Toggle Switch - eBay_v1 (Autodesk Fusion 360 design; units mm, degrees)
Autodesk Fusion 360 part; units mm, degrees
sketch "Sketch1" plane through (0, 0, 0) normal (0, 0, 1) x (1, 0, 0)
  line L0 (7.625, -14.5) -> (-7.625, -14.5)
  line L1 (-7.625, -14.5) -> (-7.625, 14.5)
  line L2 (-7.625, 14.5) -> (7.625, 14.5)
  line L3 (7.625, 14.5) -> (7.625, -14.5)
  line L4 (7.625, -14.5) -> (-7.625, 14.5) construction
  line L5 (-7.625, -14.5) -> (7.625, 14.5) construction
  circle A0 centre (0, 0) radius 5.845
  line L6 (-6.335, -5.24) -> (6.335, -5.24)
  arc A1 (6.335, -5.24) -> (6.335, -2.66) centre (6.335, -3.95) ccw
  line L7 (6.335, -2.66) -> (-6.335, -2.66)
  arc A2 (-6.335, -2.66) -> (-6.335, -5.24) centre (-6.335, -3.95) ccw
  line L8 (-7.625, -3.95) -> (7.625, -3.95) construction
  line L9 (0, 0) -> (7.625, 0) construction
  line L10 (6.335, 2.66) -> (-6.335, 2.66)
  arc A3 (-6.335, 5.24) -> (-6.335, 2.66) centre (-6.335, 3.95) ccw
  line L11 (-6.335, 5.24) -> (6.335, 5.24)
  arc A4 (6.335, 2.66) -> (6.335, 5.24) centre (6.335, 3.95) ccw
  dimension "d1" = 15.25
  dimension "d2" = 29
  dimension "d3" = 11.69
  dimension "d6" = 3.95
  dimension "d7" = 2.58
  constraint horizontal L0
  constraint perpendicular L0 L1
  constraint parallel L0 L2
  constraint parallel L1 L3
  constraint coincident L4 A0.centre
  constraint coincident L5 A0.centre
  constraint coincident A0.centre L9.start
  constraint tangent L6 A1
  constraint tangent A1 L7
  constraint parallel L6 L7
  constraint tangent L7 A2
  constraint tangent L6 A2
  constraint midpoint A2 L8.start
  constraint midpoint A1 L8.end
  constraint coincident L3 L8.end
  constraint perpendicular L3 L8
  constraint coincident L1 L8.start
  constraint midpoint L3 L9.end
  constraint symmetric L6.start L9 A3.start
  constraint symmetric L6.end L9 L11.end
  constraint symmetric A1.end L9 L10.start
  constraint symmetric L7.end L9 L10.end
  constraint symmetric A1 L9 A4
  constraint symmetric A2 L9 A3
  measures "d1" distance of L1.end L2.end
  measures "d2" distance of L0.start L2.end
  measures "d3" diameter of A0
  measures "d6" distance of A0.centre L8
  measures "d7" distance of L6 L7
extrude "Extrude1" add sketch "Sketch1" against normal blind 17.25 makes body 1
extrude "Extrude2" add sketch "Sketch1" against normal blind 2 from surface at -17.25 contours A0 L6 A1 L7 | A0 L6 L7 A2 | A0 L10 L11 A4 | A0 L10 A3 L11 | A0 L6 L7 | A0 L10 L11 bodies 1
extrude "Extrude3" add sketch "Sketch1" along normal blind 10.45 contours A0 L6 L7 | A0 L6 | A0 L7 L10 | A0 L10 L11 | A0 L11 bodies 1
thread "Thread1" "ISO Metric profile 12.0 M12x0.5 6g" major diameter 11.927 minor diameter 11.348 pitch 0.5 angle 60 resizes the face on face at (5.816, -0.582, 3.4833) on bodies 1
sketch "Sketch2" plane through (0, 0, 10.45) normal (0, 0, 1) x (-1, 0, 0)
  circle A0 centre (0, 0) radius 5.9635
  circle A1 centre (0, 0) radius 2.25
  dimension "d13" = 4.5
  constraint concentric A0 A1
  measures "d13" diameter of A1
ref_plane "WorkPlane1" through (0, 0, 27.05) normal (0, 0, 1) x (-1, 0, 0)
sketch "Sketch3" plane through (0, 0, 27.05) normal (0, 0, 1) x (1, 0, 0)
  circle A0 centre (0, 0) radius 2.96
  dimension "d15" = 5.92
  constraint coincident A0.centre origin
  measures "d15" diameter of A0
loft "Loft1" add profiles "Sketch2", "Sketch3" section 1 contours A1 section 2 separate body makes body 2
fillet "Fillet1" radius 1.5 1 edges at (-2.7597, 1.0704, 27.05) on bodies 2
move_body "Move1" bodies 2 to x (1, 0, 0) y (0, 0.976296, -0.21644) z (0, 0.21644, 0.976296) at (0, -2.2618, 0.2477)
extrude "Extrude4" add 1 faces at (0.1619, 0.6816, 10.2989) along direction (0, -0.21644, -0.976296) blind 2.5 on bodies 2 bodies 2
equation "d6 = ( 7.9 / 2 ) * 1 mm"
